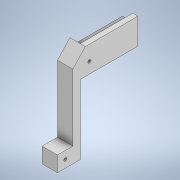
# Autodesk Inventor part: GripperServoAtt
Saved by Autodesk Inventor 2020 (Build 240168000, 168)
## iProperties
Created: 2020-01-21
Part Number: GripperServoAtt
Material: Generic
Document SubType Name: Modeling
Designer: tdmp4
Density: 1 g/cm^3
Appearance: Default
Author: tdmp4
Autodesk Inventor part; units mm, degrees
ref_plane "YZ Plane" through (0, 0, 0) normal (1, 0, 0) x (0, 1, 0)
ref_plane "XZ Plane" through (0, 0, 0) normal (0, 1, 0) x (-1, 0, 0)
ref_plane "XY Plane" through (0, 0, 0) normal (0, 0, 1) x (1, 0, 0)
sketch "Sketch1" plane through (0, 0, 0) normal (1, 0, 0) x (0, 1, 0)
  line L0 (0, 0) -> (25.4, 0)
  line L1 (25.4, 0) -> (25.4, -9.525)
  line L2 (25.4, -9.525) -> (0, -9.525)
  line L3 (0, -9.525) -> (0, 0)
  line L4 (25.4, -9.525) -> (35.5298, -9.525)
  line L5 (35.5298, -9.525) -> (35.5298, -29.845)
  line L6 (25.4, -9.525) -> (25.4, -24.4288)
  line L7 (25.4, -24.4288) -> (25.4, -29.845)
  line L8 (35.5298, -29.845) -> (26.0048, -29.845)
  line L9 (26.0048, -29.845) -> (26.0048, -80.645)
  line L10 (26.0048, -80.645) -> (35.5298, -80.645)
  line L11 (35.5298, -80.645) -> (35.5298, -29.845)
  line L12 (35.5298, -80.645) -> (41.8798, -80.645)
  line L13 (41.8798, -80.645) -> (41.8798, -15.4958)
  line L14 (41.8798, -15.4958) -> (35.5298, -15.4958)
  line L15 (35.5298, -15.4958) -> (35.5298, -80.645)
  line L16 (25.4, 0) -> (35.5298, -9.525)
  line L17 (41.8798, -15.4958) -> (35.5298, -9.525)
  line L18 (26.0048, -29.845) -> (25.4, -29.845)
  line L19 (0, 0) -> (-76.2, 0)
  line L20 (-76.2, 0) -> (-76.2, -9.525)
  line L21 (-76.2, -9.525) -> (0, -9.525)
  line L22 (0, -9.525) -> (0, 0)
  dimension "d0" = 25.4
  dimension "d1" = 9.525
  dimension "d3" = 20.32
  dimension "d11" = 50.8
  dimension "d12" = 6.35
  dimension "d13" = 76.2
  dimension "d14" = 9.525
  constraints: 46 end point, 8 parallel, 6 horizontal, 5 perpendicular, 2 vertical, 1 collinear
  measures "d0" distance of L1.end L2.end
  measures "d1" distance of L2.end L0.start
  measures "d3" distance of L4.end L5.end
  measures "d11" distance of L8.end L9.end
  measures "d12" distance of L14.end L13.end
  measures "d13" distance of L21.end L20.end
  measures "d14" distance of L19.end L20.end
extrude "Extrusion1" add sketch "Sketch1" along normal blind 19.05
sketch "Sketch4" plane through (0, 26.0048, -80.645) normal (0, -1, 0) x (1, 0, 0)
  line L0 (0, 0) -> (0, 65.1492) projected
  line L1 (19.05, 71.12) -> (19.05, 50.8) projected
  line L2 (0, 0) -> (19.05, 0)
  line L3 (19.05, 0) -> (19.05, 71.12)
  line L4 (19.05, 71.12) -> (0, 71.12)
  line L5 (0, 71.12) -> (0, 0)
  point P0 (0, 80.645)
  point P1 (0, 65.1492)
  constraints: 8 end point, 2 parallel, 1 horizontal, 1 perpendicular
extrude "Extrusion3" add sketch "Sketch4" along normal blind 16.256
sketch "Sketch5" plane through (0, 41.8798, -15.4958) normal (0, 1, 0) x (1, 0, 0)
  line L0 (0, 65.1492) -> (19.05, 65.1492) projected
  line L1 (0, 0) -> (19.05, 0) projected
  line L2 (0, 65.1492) -> (12.7, 65.1492)
  line L3 (12.7, 65.1492) -> (12.7, 0)
  line L4 (12.7, 0) -> (0, 0)
  line L5 (0, 0) -> (0, 65.1492)
  point P0 (0, -15.4958)
  dimension "d17" = 12.7
  constraints: 8 end point, 2 parallel, 1 horizontal, 1 perpendicular, 1 point on line
  measures "d17" distance of L3.end L4.end
extrude "Extrusion4" cut sketch "Sketch5" against normal blind 9.525
sketch "Sketch6" plane through (0, 0, 0) normal (-1, 0, 0) x (0, 0, 1)
  circle A0 centre (-20.3035, 23.5915) radius 1.7907
  point P0 (0, 0)
  dimension "d20" = 3.5814
  constraints: 1 centre point
  measures "d20" diameter of A0
extrude "Extrusion5" cut sketch "Sketch6" against normal blind 92.075
sketch "Sketch7" plane through (0, -76.2, 0) normal (0, 0, 1) x (1, 0, 0)
  line L0 (0, 0) -> (19.05, 0) projected
  line L1 (0, 0) -> (19.05, 0)
  line L2 (19.05, 0) -> (19.05, 19.05)
  line L3 (19.05, 19.05) -> (0, 19.05)
  line L4 (0, 19.05) -> (0, 0)
  point P0 (0, 76.2)
  dimension "d23" = 19.05
  dimension "d24" = 19.05
  constraints: 8 end point, 2 parallel, 1 horizontal, 1 perpendicular
  measures "d23" distance of L1.end L2.end
  measures "d24" distance of L2.end L3.end
extrude "Extrusion6" add sketch "Sketch7" along normal blind 19.05
sketch "Sketch8" plane through (0, 0, 0) normal (-1, 0, 0) x (0, 0, 1)
  line L0 (-9.525, -76.2) -> (19.05, -76.2) projected
  line L1 (0, -57.15) -> (19.05, -76.2)
  line L2 (19.05, -76.2) -> (19.05, -57.15)
  line L3 (19.05, -57.15) -> (0, -76.2)
  circle A0 centre (9.525, -66.675) radius 1.7907
  point P0 (0, 0)
  dimension "d27" = 3.5814
  constraints: 6 end point, 2 perpendicular, 1 centre point, 1 midpoint, 1 point on line
  measures "d27" diameter of A0
extrude "Extrusion7" cut sketch "Sketch8" against normal blind 31.75 contours A0 L1 L3 | L3 L1 A0 | L1 L3 A0 | L1 A0 L3
body "Solid1"
